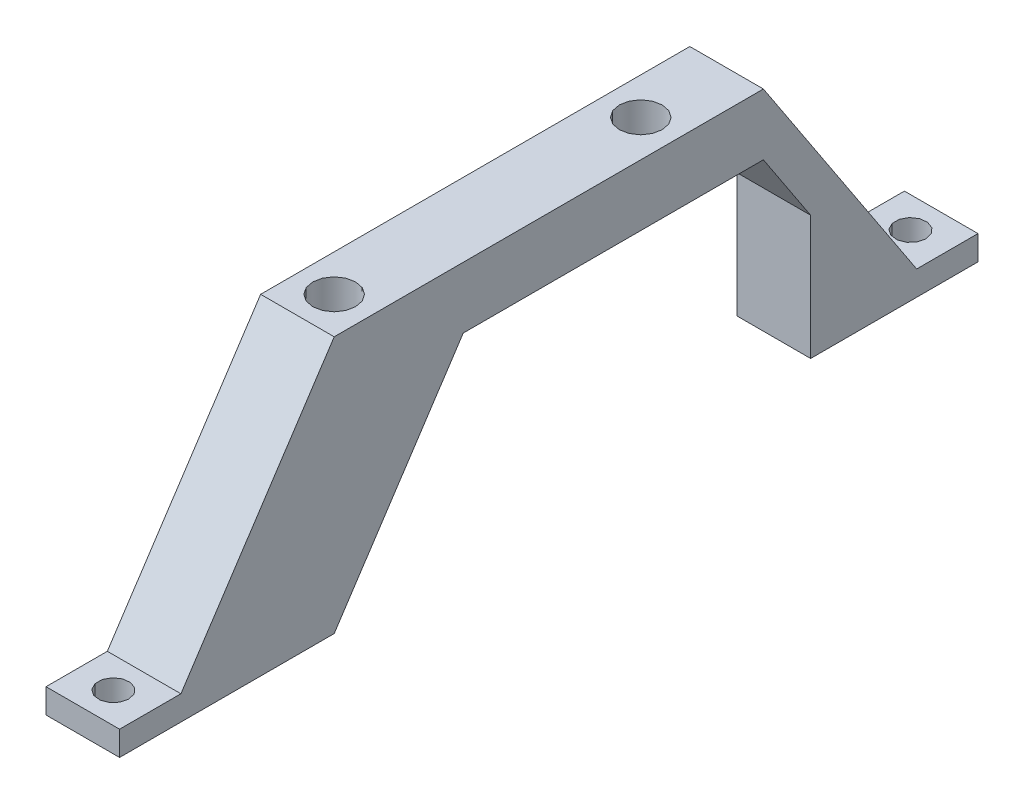
# Autodesk Inventor part: low_part_of_extrad_system
Saved by Autodesk Inventor 2025 (Build 290162000, 162)
## iProperties
Created: 2026-09-08
Part Number: low_part_of_extrad_system
Material: Типовые
Document SubType Name: Modeling
Designer: Leva
Density: 1 g/cm^3
Appearance: По умолчанию
Author: Leva
Autodesk Inventor part; units mm, degrees
ref_plane "YZ Plane" through (0, 0, 0) normal (1, 0, 0) x (0, 1, 0)
ref_plane "XZ Plane" through (0, 0, 0) normal (0, 1, 0) x (-1, 0, 0)
ref_plane "XY Plane" through (0, 0, 0) normal (0, 0, 1) x (1, 0, 0)
sketch "Эскиз1" plane through (0, 0, 0) normal (1, 0, 0) x (0, 1, 0)
  line L0 (0, 35) -> (20.96, 35) construction
  line L1 (20.96, 35) -> (20.96, -35) construction
  line L2 (20.96, -35) -> (0, -35) construction
  line L3 (0, -35) -> (0, 35) construction
  line L4 (13, 12.5) -> (0, 12.5) construction
  line L5 (0, 12.5) -> (0, -12.5) construction
  line L6 (0, -12.5) -> (13, -12.5) construction
  line L7 (13, -12.5) -> (13, 12.5) construction
  line L8 (20.96, 17.5) -> (15.96, 17.5)
  line L9 (15.96, 17.5) -> (15.96, -17.5)
  line L10 (15.96, -17.5) -> (20.96, -17.5)
  line L11 (20.96, -17.5) -> (20.96, 17.5)
  line L12 (0, 35) -> (2, 35)
  line L13 (2, 35) -> (2, 30)
  line L14 (2, 30) -> (0, 30)
  line L15 (0, 30) -> (0, 35)
  line L16 (15.96, 17.5) -> (0, 17.5)
  line L17 (0, 30) -> (0, 17.5)
  line L18 (2, 30) -> (20.96, 17.5)
  line L19 (20.96, 0) -> (0, 0) construction
  line L20 (0, -35) -> (2, -35)
  line L21 (2, -35) -> (2, -30)
  line L22 (2, -30) -> (0, -30)
  line L23 (0, -30) -> (0, -35)
  line L24 (15.96, -17.5) -> (0, -17.5)
  line L25 (0, -30) -> (0, -17.5)
  line L26 (2, -30) -> (20.96, -17.5)
  line L27 (15.96, -17.5) -> (15.96, -17.5)
  line L28 (15.96, -17.5) -> (10.1158, -21.353)
  line L29 (15.96, -17.5) -> (22.96, -17.5) construction
  line L30 (10.1158, -21.353) -> (0, -21.353)
  line L31 (0, 17.5) -> (15.96, 6.9778)
  dimension "d0" = 20.96
  dimension "d1" = 70
  dimension "d2" = 13
  dimension "d3" = 25
  dimension "d4" = 5
  dimension "d5" = 35
  dimension "d6" = 2
  dimension "d7" = 5
  dimension "d25" = 0
  dimension "d26" = 7
  constraints: 64 end point, 10 parallel, 7 perpendicular, 5 horizontal, 4 midpoint, 4 point on line, 4 symmetric about line, 1 coincident, 1 collinear, 1 equal length
  measures "d0" distance of L1.end L2.end
  measures "d1" distance of L2.end L0.start
  measures "d2" distance of L6.end L5.end
  measures "d3" distance of L5.end L4.end
  measures "d4" distance of L10.end L9.end
  measures "d5" distance of L9.end L8.end
  measures "d6" distance of L13.end L14.end
  measures "d7" distance of L12.end L13.end
  measures "d25" distance of L9.end L27.end
  measures "d26" distance of L27.end L28.end
extrude "Выдавливание1" add sketch "Эскиз1" along normal blind 6 contours L11 L10 L9 L8 | L8 L16 L17 L14 L18 | L9 L31 L16 | L26 L22 L25 L30 L28 L10 | L14 L15 L12 L13 | L21 L20 L23 L22
sketch "Эскиз2" plane through (0, 20.96, 17.5) normal (0, 1, 0) x (1, 0, 0)
  line L0 (0, 0) -> (6, 0) projected
  line L1 (3, 0) -> (3, 31) construction
  line L2 (0, 31) -> (6, 31) projected
  line L3 (3, 3) -> (3, 28) construction
  circle A0 centre (3, 3) radius 1.75
  circle A1 centre (3, 28) radius 1.75
  point P0 (0, 17.5)
  point P1 (3, 15.5)
  dimension "d10" = 25
  dimension "d11" = 3.5
  dimension "d12" = 3.5
  constraints: 4 end point, 4 midpoint, 2 centre point, 2 coincident, 1 collinear
  measures "d10" distance of L3.start L3.end
  measures "d11" diameter of A0
  measures "d12" diameter of A1
extrude "Выдавливание2" cut sketch "Эскиз2" against normal blind 4
sketch "Эскиз3" plane through (0, 2, 35) normal (0, 1, 0) x (1, 0, 0)
  line L0 (0, 0) -> (6, 0) construction
  line L1 (6, 17.5) -> (6, 5) projected
  line L2 (0, 0) -> (6, 0) construction
  line L3 (6, 0) -> (6, 5) construction
  line L4 (6, 5) -> (0, 5) construction
  line L5 (0, 5) -> (0, 0) construction
  line L6 (6, 56.353) -> (6, 70) projected
  line L7 (0, 65) -> (0, 52.5) projected
  line L8 (6, 70) -> (0, 70) construction
  line L9 (0, 70) -> (0, 65) construction
  line L10 (0, 65) -> (6, 65) construction
  line L11 (6, 65) -> (6, 70) construction
  line L12 (0, 5) -> (0, 0) construction
  line L13 (0, 2.5) -> (6, 2.5) construction
  line L14 (3, 0) -> (3, 5) construction
  line L15 (0, 67.5) -> (6, 67.5) construction
  line L16 (3, 65) -> (3, 70) construction
  circle A0 centre (3, 2.5) radius 1.25
  circle A1 centre (3, 67.5) radius 1.25
  point P0 (0, 35)
  point P1 (6, 55.5)
  dimension "d21" = 2.5
  dimension "d22" = 2.5
  constraints: 24 end point, 10 midpoint, 4 parallel, 2 centre point, 2 horizontal, 2 perpendicular
  measures "d21" diameter of A0
  measures "d22" diameter of A1
extrude "Выдавливание3" cut sketch "Эскиз3" against normal blind 2
